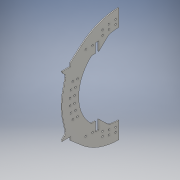
# Autodesk Inventor part: 16in outer coil
Saved by Autodesk Inventor 2016 (Build 200138000, 138)
## iProperties
Created: 2016-01-31
Part Number: 16in outer coil
Material: Polystyrene
Document SubType Name: Modeling
Designer: Scott
Density: 1.021 g/cm^3
Appearance: Smooth - White
Author: Scott
Autodesk Inventor part; units mm, degrees
ref_plane "YZ Plane" through (0, 0, 0) normal (1, 0, 0) x (0, 1, 0)
ref_plane "XZ Plane" through (0, 0, 0) normal (0, 1, 0) x (-1, 0, 0)
sketch "Sketch1" plane through (0, 0, 0) normal (1, 0, 0) x (0, 1, 0)
  arc A0 (203.2, 0) -> (-203.2, 0) centre (0, 0) ccw
  arc A1 (152.4, 0) -> (-152.4, 0) centre (0, 0) ccw
  arc A2 (185.42, 0) -> (-185.42, 0) centre (0, 0) ccw
  line L0 (0, 0) -> (152.4, 0) construction
  line L1 (0, 0) -> (220.2471, 220.2471) construction
  line L2 (0, 0) -> (-217.8171, 217.8171) construction
  line L3 (0, 0) -> (-152.4, 0) construction
  line L4 (203.2, 0) -> (418.8667, 0) construction
  line L5 (152.4, 0) -> (-185.42, 0)
  line L6 (-203.2, 0) -> (-272.3039, 0)
  line L7 (-185.42, 0) -> (-203.2, 0)
  line L8 (-152.4, 0) -> (-203.2, 0)
  line L9 (152.4, 0) -> (203.2, 0)
  arc A3 (168.91, 0) -> (-168.91, 0) centre (0, 0) ccw
  point P0 (181.5133, 37.8617)
  point P1 (184.9846, 12.7)
  point P2 (164.6231, 37.8128)
  point P3 (168.4319, 12.7)
  point P4 (174.6359, 62.3129)
  point P5 (157.0918, 62.0706)
  point P6 (37.8617, 181.5133)
  point P7 (12.7, 184.9846)
  point P8 (37.8128, 164.6231)
  point P9 (12.7, 168.4319)
  point P10 (62.3129, 174.6359)
  point P11 (62.0706, 157.0918)
  point P12 (-62.3129, 174.6359)
  point P13 (-37.8617, 181.5133)
  point P14 (-62.0706, 157.0918)
  point P15 (-37.8128, 164.6231)
  point P16 (-12.7, 168.4319)
  point P17 (-12.7, 184.9846)
  point P18 (-157.0918, 62.0706)
  point P19 (-174.6359, 62.3129)
  point P20 (-181.5133, 37.8617)
  point P21 (-164.6231, 37.8128)
  point P22 (-168.4319, 12.7)
  point P23 (-184.9846, 12.7)
  dimension "d0" = 406.4
  dimension "d2" = 304.8
  dimension "d3" = 370.84
  dimension "d5" = 50.8
  dimension "d6" = 25.4
  dimension "d7" = 25.4
  dimension "d8" = 12.7
  dimension "d9" = 12.7
  dimension "d10" = 25.4
  dimension "d11" = 25.4
  dimension "d12" = 45
  dimension "d13" = 45
  constraints: 20 end point, 16 point on circle, 12 symmetric about line, 4 centre point, 4 coincident, 3 horizontal, 3 point on line, 1 collinear
  measures "d0" diameter of A0
  measures "d2" diameter of A1
  measures "d3" diameter of A2
  measures "d5" radial gap between concentric circles of A1 A0
  measures "d6" distance of point (184.985, 12.7) point (181.513, 37.862)
  measures "d7" distance of point (168.432, 12.7) point (164.623, 37.813)
  measures "d8" distance from line of L0 point (184.985, 12.7)
  measures "d9" distance from line of L0 point (168.432, 12.7)
  measures "d10" distance of point (181.513, 37.862) point (174.636, 62.313)
  measures "d11" distance of point (164.623, 37.813) point (157.092, 62.071)
  measures "d12" angle of L3 L2
  measures "d13" angle of L0 L1
extrude "Extrusion1" add sketch "Sketch1" along normal blind 6.35 contours L9 A2 L7 A0 | L9 A3 L5 A2 | L9 A1 L5 A3
hole "Hole1" at (0, 181.5133, 37.8617) at (0, 184.9846, 12.7) at (0, 164.6231, 37.8128) at (0, 168.4319, 12.7) at (0, 174.6359, 62.3129) at (0, 157.0918, 62.0706) at (0, 62.3129, 174.6359) at (0, 37.8617, 181.5133) at (0, 62.0706, 157.0918) at (0, 37.8128, 164.6231) at (0, 12.7, 168.4319) at (0, 12.7, 184.9846) at (0, -62.0706, 157.0918) at (0, -62.3129, 174.6359) at (0, -37.8617, 181.5133) at (0, -37.8128, 164.6231) at (0, -12.7, 168.4319) at (0, -12.7, 184.9846) at (0, -184.9846, 12.7) at (0, -168.4319, 12.7) at (0, -181.5133, 37.8617) at (0, -164.6231, 37.8128) at (0, -174.6359, 62.3129) at (0, -157.0918, 62.0706) direction (1, 0, 0) diameter 6.604 end through all
sketch "Sketch2" plane through (6.35, 0, 0) normal (1, 0, 0) x (0, 0, -1)
  arc A0 (0, 215.9) -> (0, -215.9) centre (0, 0) ccw
  arc A1 (0, 203.2) -> (0, -203.2) centre (0, 0) ccw projected
  line L0 (0, 203.2) -> (0, 215.9)
  line L1 (0, -203.2) -> (0, -215.9)
  dimension "d23" = 431.8
  constraints: 4 end point, 2 point on circle, 1 centre point, 1 coincident, 1 point on line, 1 vertical
  measures "d23" diameter of A0
extrude "Extrusion2" add sketch "Sketch2" against normal blind 6.35
sketch "Sketch3" plane through (6.35, 0, 0) normal (1, 0, 0) x (0, 0, -1)
  circle A0 centre (-62.3129, -174.6359) radius 3.302 projected
  circle A1 centre (-37.8617, -181.5133) radius 3.302 projected
  circle A2 centre (-12.7, -184.9846) radius 3.302 projected
  circle A3 centre (-168.4319, -12.7) radius 3.302 projected
  circle A4 centre (-181.5133, -37.8617) radius 3.302 projected
  circle A5 centre (-157.0918, -62.0706) radius 3.302 projected
  circle A6 centre (-168.4319, 12.7) radius 3.302 projected
  circle A7 centre (-157.0918, 62.0706) radius 3.302 projected
  circle A8 centre (-174.6359, 62.3129) radius 3.302 projected
  circle A9 centre (-62.3129, 174.6359) radius 3.302 projected
  circle A10 centre (-37.8128, 164.6231) radius 3.302 projected
  circle A11 centre (-37.8617, 181.5133) radius 3.302 projected
  circle A12 centre (-12.7, 184.9846) radius 3.302 projected
  circle A13 centre (-12.7, 168.4319) radius 3.302 projected
  circle A14 centre (-62.0706, 157.0918) radius 3.302 projected
  circle A15 centre (-181.5133, 37.8617) radius 3.302 projected
  circle A16 centre (-164.6231, 37.8128) radius 3.302 projected
  circle A17 centre (-184.9846, 12.7) radius 3.302 projected
  circle A18 centre (-174.6359, -62.3129) radius 3.302 projected
  circle A19 centre (-164.6231, -37.8128) radius 3.302 projected
  circle A20 centre (-184.9846, -12.7) radius 3.302 projected
  circle A21 centre (-12.7, -168.4319) radius 3.302 projected
  circle A22 centre (-37.8128, -164.6231) radius 3.302 projected
  circle A23 centre (-62.0706, -157.0918) radius 3.302 projected
  line L0 (0, 152.4) -> (0, 215.9) projected
  arc A24 (0, 215.9) -> (0, -215.9) centre (0, 0) ccw projected
  line L1 (0, -152.4) -> (0, -215.9) projected
  arc A25 (0, 152.4) -> (0, -152.4) centre (0, 0) ccw projected
extrude "Extrusion3" cut sketch "Sketch3" against normal blind 3.175
sketch "Sketch4" plane through (3.175, 0, 0) normal (1, 0, 0) x (0, 0, -1)
  arc A0 (0, 215.9) -> (0, -215.9) centre (0, 0) ccw projected
  line L0 (-183.162, -114.3) -> (-266.6206, -114.3)
  line L1 (-183.162, -114.3) -> (-183.162, -127)
  line L2 (-183.162, -127) -> (-174.5961, -127)
  arc A1 (-183.162, -114.3) -> (-174.5961, -127) centre (0, 0) ccw
  line L3 (0, 0) -> (-55.1086, 0) construction
  line L4 (-183.162, 114.3) -> (-183.162, 127)
  line L5 (-183.162, 127) -> (-174.5961, 127)
  arc A2 (-174.5961, 127) -> (-183.162, 114.3) centre (0, 0) ccw
  line L6 (-183.162, -127) -> (-141.3083, -163.2323)
  line L7 (-141.3083, -163.2323) -> (-141.3083, -138.6282)
  line L8 (-141.3083, -138.6282) -> (-174.5961, -127)
  line L9 (-183.162, 127) -> (-141.3083, 163.2323)
  line L10 (-174.5961, 127) -> (-141.3083, 120.9425)
  line L11 (-141.3083, 120.9425) -> (-141.3083, 163.2323)
  dimension "d28" = 114.3
  dimension "d29" = 12.7
  constraints: 24 end point, 8 point on circle, 3 horizontal, 3 symmetric about line, 2 centre point, 2 tangent, 2 vertical, 1 concentric, 1 other
  measures "d28" distance from line of point (0, 0) L0
  measures "d29" distance of L0.start L1.end
extrude "Extrusion5" add sketch "Sketch4" against normal blind 3.175 contours L11 L10 A0 | A0 L5 L9 | A0 L2 L1 | A0 L4 L5 | A0 L6 L2
sketch "Sketch5" plane through (3.175, 0, 0) normal (1, 0, 0) x (0, 0, -1)
  line L0 (-183.162, 127) -> (-183.162, 114.3) projected
  line L1 (-183.162, 114.3) -> (-195.862, 114.3)
  line L2 (-195.862, 114.3) -> (-210.8216, 46.5518)
  arc A0 (-183.162, 114.3) -> (-183.162, -114.3) centre (0, 0) ccw projected
  line L3 (-210.8216, 46.5518) -> (-192.3409, 71.251)
  line L4 (-192.3409, 71.251) -> (-183.162, 114.3)
  line L5 (-183.162, -127) -> (-183.162, -114.3) projected
  line L6 (-183.162, -114.3) -> (-195.862, -114.3)
  line L7 (-195.862, -114.3) -> (-210.8216, -46.5518)
  line L8 (-210.8216, -46.5518) -> (-195.3713, -59.0073)
  line L9 (-195.3713, -59.0073) -> (-183.162, -114.3)
  dimension "d34" = 12.7
  dimension "d35" = 12.7
  constraints: 16 end point, 2 horizontal, 2 point on circle, 2 tangent, 1 parallel, 1 point on line
  measures "d34" distance of L0.end L1.end
  measures "d35" distance of L5.end L6.end
extrude "Extrusion6" add sketch "Sketch5" against normal blind 3.175 contours A0 L2 L1 | A0 L6 L7
sketch "Sketch9" plane through (3.175, 0, 0) normal (1, 0, 0) x (0, 0, -1)
  line L0 (-92.2547, 269.24) -> (-92.2547, 299.72) projected
  line L1 (-150.1234, 299.72) -> (-92.2547, 299.72) projected
  line L2 (-198.5102, 285.4918) -> (-150.1234, 299.72) projected
  arc A0 (-198.5102, 285.4918) -> (-213.4606, 273.6152) centre (-191.3446, 261.1234) ccw projected
  line L3 (-215.9318, 269.24) -> (-213.4606, 273.6152) projected
  line L4 (-92.2547, 269.24) -> (-215.9318, 269.24) projected
  circle A1 centre (-125.6507, 284.48) radius 3.302 projected
  circle A2 centre (-100.2507, 284.48) radius 3.302 projected
  arc A3 (-60.2763, 194.0541) -> (60.2763, -194.0541) centre (0, 0) ccw projected
  line L5 (-92.2547, -15.24) -> (-92.2547, 15.24) projected
  line L6 (-92.2547, 15.24) -> (-215.9318, 15.24) projected
  line L7 (-215.9318, 15.24) -> (-213.4606, 10.8648) projected
  arc A4 (-213.4606, 10.8648) -> (-198.5102, -1.0118) centre (-191.3446, 23.3566) ccw projected
  line L8 (-198.5102, -1.0118) -> (-150.1234, -15.24) projected
  line L9 (-150.1234, -15.24) -> (-92.2547, -15.24) projected
  circle A5 centre (-100.2507, 0) radius 3.302 projected
  circle A6 centre (-125.6507, 0) radius 3.302 projected
  line L10 (-92.2547, 127) -> (-92.2547, 157.48) projected
  line L11 (-150.1234, 157.48) -> (-92.2547, 157.48) projected
  line L12 (-198.5102, 143.2518) -> (-150.1234, 157.48) projected
  arc A7 (-198.5102, 143.2518) -> (-213.4606, 131.3752) centre (-191.3446, 118.8834) ccw projected
  line L13 (-215.9318, 127) -> (-213.4606, 131.3752) projected
  line L14 (-92.2547, 127) -> (-215.9318, 127) projected
  circle A8 centre (-125.6507, 142.24) radius 3.302 projected
  circle A9 centre (-100.2507, 142.24) radius 3.302 projected
  line L15 (-92.2547, -157.48) -> (-92.2547, -127) projected
  line L16 (-92.2547, -127) -> (-215.9318, -127) projected
  line L17 (-215.9318, -127) -> (-213.4606, -131.3752) projected
  arc A10 (-213.4606, -131.3752) -> (-198.5102, -143.2518) centre (-191.3446, -118.8834) ccw projected
  line L18 (-198.5102, -143.2518) -> (-150.1234, -157.48) projected
  line L19 (-150.1234, -157.48) -> (-92.2547, -157.48) projected
  circle A11 centre (-100.2507, -142.24) radius 3.302 projected
  circle A12 centre (-125.6507, -142.24) radius 3.302 projected
  point P0 (0, 0)
  constraints: 4 coincident
hole "Hole4" at (3.175, 142.24, 100.2507) at (3.175, 142.24, 125.6507) at (3.175, -142.24, 100.2507) at (3.175, -142.24, 125.6507) direction (-1, 0, 0) diameter 6.604 end through all
sketch "Sketch11" plane through (3.175, 0, 0) normal (1, 0, 0) x (0, 0, -1)
  line L0 (-88.9, -145.9119) -> (-88.9, -103.2908) projected
  line L1 (-76.2, -103.2908) -> (-76.2, -145.9119) projected
  line L2 (-88.9, 103.2908) -> (-88.9, 145.9119) projected
  line L3 (-76.2, 145.9119) -> (-76.2, 103.2908) projected
  line L4 (-88.9, 145.9119) -> (-76.2, 145.9119)
  line L5 (-76.2, 145.9119) -> (-76.2, 103.2908)
  line L6 (-76.2, 103.2908) -> (-88.9, 103.2908)
  line L7 (-88.9, 103.2908) -> (-88.9, 145.9119)
  line L8 (-88.9, -145.9119) -> (-76.2, -145.9119)
  line L9 (-76.2, -145.9119) -> (-76.2, -103.2908)
  line L10 (-76.2, -103.2908) -> (-88.9, -103.2908)
  line L11 (-88.9, -103.2908) -> (-88.9, -145.9119)
  point P0 (0, 0)
  constraints: 16 end point, 4 parallel, 2 horizontal, 2 perpendicular
extrude "Extrusion10" cut sketch "Sketch11" against normal blind 25.4
sketch "Sketch12" plane through (3.175, 0, 0) normal (1, 0, 0) x (0, 0, -1)
  circle A0 centre (-62.0706, -157.0918) radius 3.302 projected
  circle A1 centre (-37.8128, -164.6231) radius 3.302 projected
  circle A2 centre (-12.7, -168.4319) radius 3.302 projected
  circle A3 centre (-184.9846, -12.7) radius 3.302 projected
  circle A4 centre (-164.6231, -37.8128) radius 3.302 projected
  circle A5 centre (-174.6359, -62.3129) radius 3.302 projected
  circle A6 centre (-184.9846, 12.7) radius 3.302 projected
  circle A7 centre (-164.6231, 37.8128) radius 3.302 projected
  circle A8 centre (-181.5133, 37.8617) radius 3.302 projected
  circle A9 centre (-62.0706, 157.0918) radius 3.302 projected
  circle A10 centre (-12.7, 168.4319) radius 3.302 projected
  circle A11 centre (-12.7, 184.9846) radius 3.302 projected
  circle A12 centre (-37.8617, 181.5133) radius 3.302 projected
  circle A13 centre (-37.8128, 164.6231) radius 3.302 projected
  circle A14 centre (-62.3129, 174.6359) radius 3.302 projected
  circle A15 centre (-174.6359, 62.3129) radius 3.302 projected
  circle A16 centre (-157.0918, 62.0706) radius 3.302 projected
  circle A17 centre (-168.4319, 12.7) radius 3.302 projected
  circle A18 centre (-157.0918, -62.0706) radius 3.302 projected
  circle A19 centre (-181.5133, -37.8617) radius 3.302 projected
  circle A20 centre (-168.4319, -12.7) radius 3.302 projected
  circle A21 centre (-12.7, -184.9846) radius 3.302 projected
  circle A22 centre (-37.8617, -181.5133) radius 3.302 projected
  circle A23 centre (-62.3129, -174.6359) radius 3.302 projected
  line L0 (-76.2, -131.9823) -> (-76.2, -145.9119) projected
  line L1 (-76.2, -145.9119) -> (-88.9, -145.9119) projected
  line L2 (-88.9, -145.9119) -> (-88.9, -123.7843) projected
  arc A24 (-88.9, 123.7843) -> (-88.9, -123.7843) centre (0, 0) ccw projected
  line L3 (-88.9, 123.7843) -> (-88.9, 145.9119) projected
  line L4 (-88.9, 145.9119) -> (-76.2, 145.9119) projected
  line L5 (-76.2, 145.9119) -> (-76.2, 131.9823) projected
  arc A25 (0, 152.4) -> (-76.2, 131.9823) centre (0, 0) ccw projected
  line L6 (0, 215.9) -> (0, 152.4) projected
  arc A26 (0, 215.9) -> (-141.3083, 163.2323) centre (0, 0) ccw projected
  line L7 (-141.3083, 163.2323) -> (-183.162, 127) projected
  line L8 (-183.162, 127) -> (-183.162, 114.3) projected
  line L9 (-183.162, 114.3) -> (-195.862, 114.3) projected
  line L10 (-195.862, 114.3) -> (-210.8216, 46.5518) projected
  arc A27 (-210.8216, 46.5518) -> (-210.8216, -46.5518) centre (0, 0) ccw projected
  line L11 (-210.8216, -46.5518) -> (-195.862, -114.3) projected
  line L12 (-195.862, -114.3) -> (-183.162, -114.3) projected
  line L13 (-183.162, -114.3) -> (-183.162, -127) projected
  line L14 (-183.162, -127) -> (-141.3083, -163.2323) projected
  arc A28 (-141.3083, -163.2323) -> (0, -215.9) centre (0, 0) ccw projected
  line L15 (0, -152.4) -> (0, -215.9) projected
  arc A29 (-76.2, -131.9823) -> (0, -152.4) centre (0, 0) ccw projected
  circle A30 centre (-125.6507, -142.24) radius 3.302 projected
  circle A31 centre (-125.6507, 142.24) radius 3.302 projected
  circle A32 centre (-100.2507, 142.24) radius 3.302 projected
  circle A33 centre (-100.2507, -142.24) radius 3.302 projected
  line L16 (-76.2, -103.2908) -> (-76.2, -145.9119) projected
  line L17 (-76.2, 145.9119) -> (-76.2, 103.2908) projected
  line L18 (-76.2, -131.9823) -> (-76.2, -145.9119) projected
  line L19 (-76.2, -145.9119) -> (-76.2, -123.8289)
  arc A34 (-76.2, -131.9823) -> (0, -152.4) centre (0, 0) ccw projected
  line L20 (-249.0244, -114.3) -> (0, -114.3) projected
  line L21 (-76.2, -131.9823) -> (-76.2, -123.8289)
  arc A35 (-76.2, -131.9823) -> (-38.1, -147.5607) centre (0, 0) ccw
  arc A36 (0, 152.4) -> (-76.2, 131.9823) centre (0, 0) ccw projected
  line L22 (0, 0) -> (-39.444, 0)
  line L23 (-249.0244, 127) -> (0, 127)
  line L24 (-76.2, 145.9119) -> (-76.2, 131.9823) projected
  line L25 (-76.2, 127) -> (-76.2, 131.9823)
  arc A37 (-38.1, 147.5607) -> (-76.2, 131.9823) centre (0, 0) ccw
  line L26 (-249.0244, 123.825) -> (0, 123.825)
  line L27 (-249.0244, -114.3) -> (0, -114.3)
  line L28 (-76.2, 123.825) -> (-38.1, 147.5607)
  line L29 (0, -123.825) -> (-249.0244, -123.825)
  line L30 (-76.2, -123.8289) -> (-38.1, -147.5607)
  dimension "d67" = 22.1276
  dimension "d68" = 38.1
  dimension "d71" = 38.1
  dimension "d72" = 8.1573
  dimension "d74" = 8.1534
  constraints: 20 end point, 8 point on circle, 5 horizontal, 5 point on line, 2 centre point, 2 vertical, 8 other
  measures "d67" distance of L1.end L2.end
  measures "d68" distance from line of L16 L30.end
  measures "d71" distance from line of L5 L28.end
  measures "d72" distance of L5.end L28.start
  measures "d74" distance of L0.start L19.end
extrude "Extrusion11" add sketch "Sketch12" against normal blind 3.175 contours L16 L30 A29 | L17 L23 L28 | L17 A25 L28 L23
sketch "Sketch13" plane through (3.175, 0, 0) normal (1, 0, 0) x (0, 0, -1)
  circle A0 centre (-62.0706, -157.0918) radius 3.302 projected
  circle A1 centre (-37.8128, -164.6231) radius 3.302 projected
  circle A2 centre (-12.7, -168.4319) radius 3.302 projected
  circle A3 centre (-184.9846, -12.7) radius 3.302 projected
  circle A4 centre (-164.6231, -37.8128) radius 3.302 projected
  circle A5 centre (-174.6359, -62.3129) radius 3.302 projected
  circle A6 centre (-184.9846, 12.7) radius 3.302 projected
  circle A7 centre (-164.6231, 37.8128) radius 3.302 projected
  circle A8 centre (-181.5133, 37.8617) radius 3.302 projected
  circle A9 centre (-62.0706, 157.0918) radius 3.302 projected
  circle A10 centre (-12.7, 168.4319) radius 3.302 projected
  circle A11 centre (-12.7, 184.9846) radius 3.302 projected
  circle A12 centre (-37.8617, 181.5133) radius 3.302 projected
  circle A13 centre (-37.8128, 164.6231) radius 3.302 projected
  circle A14 centre (-62.3129, 174.6359) radius 3.302 projected
  circle A15 centre (-174.6359, 62.3129) radius 3.302 projected
  circle A16 centre (-157.0918, 62.0706) radius 3.302 projected
  circle A17 centre (-168.4319, 12.7) radius 3.302 projected
  circle A18 centre (-157.0918, -62.0706) radius 3.302 projected
  circle A19 centre (-181.5133, -37.8617) radius 3.302 projected
  circle A20 centre (-168.4319, -12.7) radius 3.302 projected
  circle A21 centre (-12.7, -184.9846) radius 3.302 projected
  circle A22 centre (-37.8617, -181.5133) radius 3.302 projected
  circle A23 centre (-62.3129, -174.6359) radius 3.302 projected
  line L0 (-76.2, -123.8289) -> (-76.2, -145.9119) projected
  line L1 (-76.2, -145.9119) -> (-88.9, -145.9119) projected
  line L2 (-88.9, -145.9119) -> (-88.9, -123.7843) projected
  arc A24 (-88.9, 123.7843) -> (-88.9, -123.7843) centre (0, 0) ccw projected
  line L3 (-88.9, 123.7843) -> (-88.9, 145.9119) projected
  line L4 (-88.9, 145.9119) -> (-76.2, 145.9119) projected
  line L5 (-76.2, 145.9119) -> (-76.2, 123.825) projected
  line L6 (-76.2, 123.825) -> (-38.1, 147.5607) projected
  arc A25 (0, 152.4) -> (-38.1, 147.5607) centre (0, 0) ccw projected
  line L7 (0, 215.9) -> (0, 152.4) projected
  arc A26 (0, 215.9) -> (-141.3083, 163.2323) centre (0, 0) ccw projected
  line L8 (-141.3083, 163.2323) -> (-183.162, 127) projected
  line L9 (-183.162, 127) -> (-183.162, 114.3) projected
  line L10 (-183.162, 114.3) -> (-195.862, 114.3) projected
  line L11 (-195.862, 114.3) -> (-210.8216, 46.5518) projected
  arc A27 (-210.8216, 46.5518) -> (-210.8216, -46.5518) centre (0, 0) ccw projected
  line L12 (-210.8216, -46.5518) -> (-195.862, -114.3) projected
  line L13 (-195.862, -114.3) -> (-183.162, -114.3) projected
  line L14 (-183.162, -114.3) -> (-183.162, -127) projected
  line L15 (-183.162, -127) -> (-141.3083, -163.2323) projected
  arc A28 (-141.3083, -163.2323) -> (0, -215.9) centre (0, 0) ccw projected
  line L16 (0, -152.4) -> (0, -215.9) projected
  arc A29 (-38.1, -147.5607) -> (0, -152.4) centre (0, 0) ccw projected
  line L17 (-38.1, -147.5607) -> (-76.2, -123.8289) projected
  circle A30 centre (-125.6507, -142.24) radius 3.302 projected
  circle A31 centre (-125.6507, 142.24) radius 3.302 projected
  circle A32 centre (-100.2507, 142.24) radius 3.302 projected
  circle A33 centre (-100.2507, -142.24) radius 3.302 projected
  line L18 (-76.2, -123.8289) -> (-76.2, -111.1289)
  arc A34 (-88.9, 123.7843) -> (-88.9, -123.7843) centre (0, 0) ccw projected
  line L19 (-88.9, 123.7843) -> (-88.9, -111.0843)
  line L20 (-88.9, -145.9119) -> (-88.9, -123.7843) projected
  line L21 (-88.9, -123.7843) -> (-88.9, -111.0843)
  line L22 (-88.9, -111.0843) -> (-104.3362, -111.0843)
  line L23 (-76.2, -123.8289) -> (-38.1, -147.5607) projected
  line L24 (-76.2, -111.1289) -> (-38.1, -147.5607)
  line L25 (-76.2, -111.1289) -> (-88.9, -111.0843)
  arc A35 (-104.3362, -111.0843) -> (-88.9, -123.7843) centre (0, 0) ccw
  line L26 (-76.2, -123.8289) -> (-38.1, -147.5607)
  dimension "d78" = 12.7
  dimension "d79" = 12.7
  dimension "d81" = 38.1
  constraints: 14 end point, 4 point on circle, 3 collinear, 1 centre point, 1 perpendicular, 1 vertical
  measures "d78" distance of L0.start L18.end
  measures "d79" distance of L2.end L19.end
  measures "d81" horizontal distance of L18.end L17.start
extrude "Extrusion12" add sketch "Sketch13" against normal blind 3.175 contours L18 L24 L17 | L21 A24 L22
ref_plane "Work Plane1" through (3.175, 0, 88.9) normal (0, 1, 0) x (1, 0, 0)
mirror "Mirror1" about plane through (3.175, 0, 88.9) normal (0, 1, 0) of "Extrusion12"
fillet "Fillet1" radius 12.7 4 edges at (1.5875, -111.0843, 104.3362) (1.5875, 111.0843, 104.3362) (1.5875, -147.5607, 38.1) (1.5875, 147.5607, 38.1)
sketch "Sketch14" plane through (3.175, 0, 0) normal (1, 0, 0) x (0, 0, -1)
  arc A0 (0, 152.4) -> (-34.6616, 148.406) centre (0, 0) ccw projected
  line L0 (0, 215.9) -> (0, 152.4) projected
  arc A1 (0, 215.9) -> (-141.3083, 163.2323) centre (0, 0) ccw projected
  line L1 (-141.3083, 163.2323) -> (-183.162, 127) projected
  line L2 (-183.162, 127) -> (-183.162, 114.3) projected
  line L3 (-183.162, 114.3) -> (-195.862, 114.3) projected
  line L4 (-195.862, 114.3) -> (-210.8216, 46.5518) projected
  arc A2 (-210.8216, 46.5518) -> (-210.8216, -46.5518) centre (0, 0) ccw projected
  line L5 (-210.8216, -46.5518) -> (-195.862, -114.3) projected
  line L6 (-195.862, -114.3) -> (-183.162, -114.3) projected
  line L7 (-183.162, -114.3) -> (-183.162, -127) projected
  line L8 (-183.162, -127) -> (-141.3083, -163.2323) projected
  arc A3 (-141.3083, -163.2323) -> (0, -215.9) centre (0, 0) ccw projected
  line L9 (0, -152.4) -> (0, -215.9) projected
  arc A4 (-34.6616, -148.406) -> (0, -152.4) centre (0, 0) ccw projected
  arc A5 (-40.5502, -145.2178) -> (-34.6616, -148.406) centre (-31.7731, -136.0388) ccw projected
  line L10 (-40.5502, -145.2178) -> (-76.2, -111.1289) projected
  line L11 (-76.2, -111.1289) -> (-76.2, -145.9119) projected
  line L12 (-76.2, -145.9119) -> (-88.9, -145.9119) projected
  line L13 (-88.9, -145.9119) -> (-88.9, -111.0843) projected
  line L14 (-88.9, -111.0843) -> (-99.1797, -111.0843) projected
  arc A6 (-108.1961, -107.3283) -> (-99.1797, -111.0843) centre (-99.1797, -98.3843) ccw projected
  arc A7 (-108.1961, 107.3283) -> (-108.1961, -107.3283) centre (0, 0) ccw projected
  arc A8 (-99.1797, 111.0843) -> (-108.1961, 107.3283) centre (-99.1797, 98.3843) ccw projected
  line L15 (-88.9, 111.0843) -> (-99.1797, 111.0843) projected
  line L16 (-88.9, 111.0843) -> (-88.9, 145.9119) projected
  line L17 (-88.9, 145.9119) -> (-76.2, 145.9119) projected
  line L18 (-76.2, 145.9119) -> (-76.2, 111.1289) projected
  line L19 (-40.5502, 145.2178) -> (-76.2, 111.1289) projected
  arc A9 (-34.6616, 148.406) -> (-40.5502, 145.2178) centre (-31.7731, 136.0388) ccw projected
  circle A10 centre (-62.0706, -157.0918) radius 3.302 projected
  circle A11 centre (-37.8128, -164.6231) radius 3.302 projected
  circle A12 centre (-12.7, -168.4319) radius 3.302 projected
  circle A13 centre (-184.9846, -12.7) radius 3.302 projected
  circle A14 centre (-164.6231, -37.8128) radius 3.302 projected
  circle A15 centre (-174.6359, -62.3129) radius 3.302 projected
  circle A16 centre (-184.9846, 12.7) radius 3.302 projected
  circle A17 centre (-164.6231, 37.8128) radius 3.302 projected
  circle A18 centre (-181.5133, 37.8617) radius 3.302 projected
  circle A19 centre (-62.0706, 157.0918) radius 3.302 projected
  circle A20 centre (-12.7, 168.4319) radius 3.302 projected
  circle A21 centre (-12.7, 184.9846) radius 3.302 projected
  circle A22 centre (-37.8617, 181.5133) radius 3.302 projected
  circle A23 centre (-37.8128, 164.6231) radius 3.302 projected
  circle A24 centre (-62.3129, 174.6359) radius 3.302 projected
  circle A25 centre (-174.6359, 62.3129) radius 3.302 projected
  circle A26 centre (-157.0918, 62.0706) radius 3.302 projected
  circle A27 centre (-168.4319, 12.7) radius 3.302 projected
  circle A28 centre (-157.0918, -62.0706) radius 3.302 projected
  circle A29 centre (-181.5133, -37.8617) radius 3.302 projected
  circle A30 centre (-168.4319, -12.7) radius 3.302 projected
  circle A31 centre (-12.7, -184.9846) radius 3.302 projected
  circle A32 centre (-37.8617, -181.5133) radius 3.302 projected
  circle A33 centre (-62.3129, -174.6359) radius 3.302 projected
  circle A34 centre (-125.6507, -142.24) radius 3.302 projected
  circle A35 centre (-125.6507, 142.24) radius 3.302 projected
  circle A36 centre (-100.2507, 142.24) radius 3.302 projected
  circle A37 centre (-100.2507, -142.24) radius 3.302 projected
  line L20 (-183.162, 114.3) -> (-183.162, 127) projected
  line L21 (-183.162, 120.65) -> (-194.4599, 120.65)
  line L22 (-92.2547, 127) -> (-92.2547, 157.48) projected
  line L23 (-150.1234, 157.48) -> (-92.2547, 157.48) projected
  line L24 (-198.5102, 143.2518) -> (-150.1234, 157.48) projected
  arc A38 (-198.5102, 143.2518) -> (-213.4606, 131.3752) centre (-191.3446, 118.8834) ccw projected
  line L25 (-215.9318, 127) -> (-213.4606, 131.3752) projected
  line L26 (-92.2547, 127) -> (-215.9318, 127) projected
  circle A39 centre (-125.6507, 142.24) radius 3.302 projected
  circle A40 centre (-100.2507, 142.24) radius 3.302 projected
  arc A41 (-213.4606, 109.9248) -> (-199.3896, 98.3243) centre (-191.3446, 122.4166) ccw
  line L27 (-215.9318, 114.3) -> (-213.4606, 109.9248)
  line L28 (-210.8216, 46.5518) -> (-195.862, 114.3) projected
  line L29 (-199.3896, 98.3243) -> (-195.862, 114.3)
  line L30 (-195.862, 114.3) -> (-215.9318, 114.3)
  arc A42 (-108.1961, 107.3283) -> (-108.1961, -107.3283) centre (0, 0) ccw projected
  line L31 (-152.4, 0) -> (-174.3168, 0)
  line L32 (-195.862, -114.3) -> (-199.3896, -98.3243)
  arc A43 (-199.3896, -98.3243) -> (-213.4606, -109.9248) centre (-191.3446, -122.4166) ccw
  line L33 (-195.862, -114.3) -> (-215.9318, -114.3)
  line L34 (-213.4606, -109.9248) -> (-215.9318, -114.3)
  line L35 (-199.3896, -98.3243) -> (-210.8216, -46.5518)
  constraints: 16 end point, 7 symmetric about line, 4 point on circle, 3 horizontal, 1 collinear, 1 midpoint, 1 point on line, 2 other
extrude "Extrusion13" add sketch "Sketch14" against normal blind 3.175 contours L5 L33 L34 A43
mirror "Mirror2" about plane through (3.175, 0, 88.9) normal (0, 1, 0) of "Extrusion13"
fillet "Fillet2" radius 12.7 2 edges at (1.5875, 98.3243, 199.3896) (1.5875, -98.3243, 199.3896)
sketch "Sketch15" plane through (3.175, 0, 0) normal (1, 0, 0) x (0, 0, -1)
  point P0 (0, 0)
body "Solid1"
